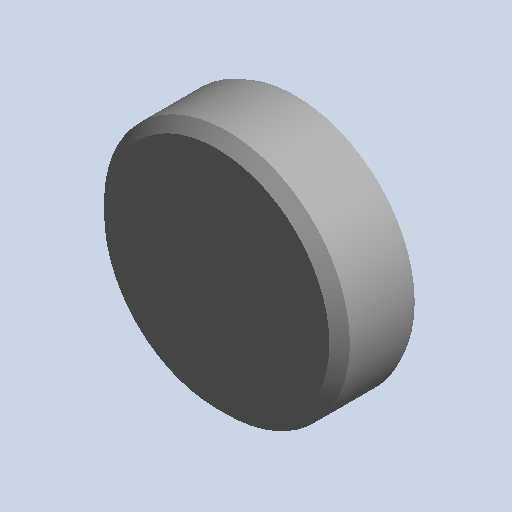
# Autodesk Inventor part: LIdar_p2
Saved by Autodesk Inventor 2026 (Build 300175050, 175E)
## iProperties
Part Number: LIdar_p2
Material: Generic
Document SubType Name: Modeling
Designer: Kartik
Mass: 92.2089 g
Surface Area: 129.237 cm^2
Volume: 92.2089 cm^3
Density: 1 g/cm^3
Appearance: Default
Author: Kartik
Autodesk Inventor part; units mm, degrees
ref_plane "YZ Plane" through (0, 0, 0) normal (1, 0, 0) x (0, 1, 0)
ref_plane "XZ Plane" through (0, 0, 0) normal (0, 1, 0) x (-1, 0, 0)
ref_plane "XY Plane" through (0, 0, 0) normal (0, 0, 1) x (1, 0, 0)
sketch "Sketch1" plane through (0, 0, 0) normal (0, 0, 1) x (1, 0, 0)
  circle A0 centre (0, 0) radius 35
  dimension "d0" = 70
  constraints: 1 centre point, 1 coincident
  measures "d0" diameter of A0
extrude "Extrusion1" add sketch "Sketch1" along normal blind 2
sketch "Sketch2" plane through (0, 0, 2) normal (0, 0, 1) x (1, 0, 0)
  circle A0 centre (0, 0) radius 36
  dimension "d3" = 72
  constraints: 1 centre point, 1 coincident
  measures "d3" diameter of A0
extrude "Extrusion2" add sketch "Sketch2" along normal blind 21
chamfer "Chamfer1" distance 3 angle 45 1 edges at (-36, 0, 23)
body "Solid1"
